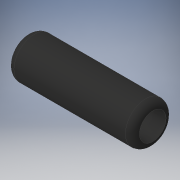
# Autodesk Inventor part: 5.5 Sleeve Handle
Saved by Autodesk Inventor 2017 (Build 210142000, 142)
## iProperties
Created: 2020-02-04
Part Number: 5.5 Sleeve Handle
Material: Rubber
Document SubType Name: Modeling
Designer: 10042265
Density: 0.93 g/cm^3
Appearance: Rubber - Black
Author: 10042265
Autodesk Inventor part; units mm, degrees
ref_plane "YZ Plane" through (0, 0, 0) normal (1, 0, 0) x (0, 1, 0)
ref_plane "XZ Plane" through (0, 0, 0) normal (0, 1, 0) x (-1, 0, 0)
ref_plane "XY Plane" through (0, 0, 0) normal (0, 0, 1) x (1, 0, 0)
sketch "Sketch3" plane through (0, 0, 0) normal (0, 0, 1) x (1, 0, 0)
  line L0 (0, 0) -> (113.5126, 0)
  line L1 (113.5126, 0) -> (113.5126, 6.35)
  line L2 (113.5126, 6.35) -> (3.9624, 6.35)
  line L3 (3.9624, 6.35) -> (3.9624, 17.4625)
  line L4 (3.9624, 17.4625) -> (0, 17.4625)
  line L5 (0, 17.4625) -> (0, 0)
  line L6 (0, 17.4625) -> (0, 18.415) construction
  line L7 (0, 18.415) -> (113.5126, 18.415) construction
  line L8 (113.5126, 18.415) -> (113.5126, 0) construction
  dimension "d163" = 113.5126
  dimension "d164" = 6.35
  dimension "d165" = 109.5502
  dimension "d166" = 11.1125
  dimension "d167" = 0.9525
  constraints: 18 end point, 7 perpendicular, 2 horizontal
  measures "d163" distance of L0.start L0.end
  measures "d164" distance of L0.end L1.end
  measures "d165" distance of L1.end L2.end
  measures "d166" distance of L2.end L3.end
  measures "d167" distance of L4.end L6.end
revolve "Revolution2" add sketch "Sketch3" angle 360 about axis through (0, 18.415, 0) along (1, 0, 0)
fillet "Fillet1" radius 6.35 1 edges at (0, 36.83, 0)
fillet "Fillet2" radius 6.35 1 edges at (113.5126, 36.83, 0)
body "Solid2"
